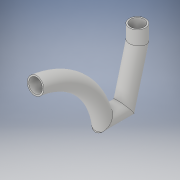
# Autodesk Inventor part: test_01
Saved by Autodesk Inventor 2019 (Build 230136000, 136)
## iProperties
Created: 2020-10-27
Part Number: test_01
Material: Genérico
Document SubType Name: Modeling
Designer: Juan M. Casillas
Density: 1 g/cm^3
Appearance: Valor por defecto
Author: Juan M. Casillas
## iProperties of the stored document test_01_3DPrint.ipt
Created: 2020-10-27
Part Number: test_01_3DPrint
Material: Genérico
Document SubType Name: Modeling
Designer: Juan M. Casillas
Density: 1 g/cm^3
Appearance: Valor por defecto
Author: Juan M. Casillas
Autodesk Inventor part; units mm, degrees
ref_plane "YZ Plane" through (0, 0, 0) normal (1, 0, 0) x (0, 1, 0)
ref_plane "XZ Plane" through (0, 0, 0) normal (0, 1, 0) x (-1, 0, 0)
ref_plane "XY Plane" through (0, 0, 0) normal (0, 0, 1) x (1, 0, 0)
sketch "Sketch7" plane through (0, 0, 0) normal (1, 0, 0) x (0, 1, 0)
  line L0 (0, 0) -> (0, 44) construction
  line L1 (0, 0) -> (44, 0) construction
  line L2 (44, 0) -> (44, 44) construction
  line L3 (44, 44) -> (0, 44) construction
  arc A0 (0, 0) -> (44, 44) centre (-6.9929, 50.9929) ccw
  line L4 (0, 0) -> (0, -22.5)
  line L5 (0, -22.5) -> (39.6996, -33.1375)
  line L6 (0, -22.5) -> (41.1, -22.5) construction
  line L7 (39.6996, -33.1375) -> (50.6736, -33.1375)
  dimension "d15" = 44
  dimension "d16" = 44
  dimension "d17" = 22.5
  dimension "d19" = 41.1
  dimension "d20" = 15
  dimension "d21" = 10.974
  constraints: 16 end point, 3 horizontal, 2 perpendicular, 2 point on circle, 2 vertical, 1 centre point, 1 equal length
  measures "d15" distance of L0.start L0.end
  measures "d16" distance of L0.start L1.end
  measures "d17" distance of L0.start L4.end
  measures "d19" distance of L4.end L5.end
  measures "d20" angle of L5 L6
  measures "d21" distance of L5.end L7.end
sketch "Sketch8" plane through (0, 0, 0) normal (0, 0, 1) x (1, 0, 0)
  line L0 (-43.2276, 7.3965) -> (-33.2276, 7.3952)
  line L1 (-33.2276, 7.3952) -> (-38.2287, -1.2644)
  line L2 (-38.2287, -1.2644) -> (-43.2276, 7.3965)
  circle A0 centre (-38.2279, 4.5091) radius 5.7817
  point P0 (0, 0)
  dimension "d18" = 10
  constraints: 6 end point, 1 centre point, 1 coincident, 7 other
  measures "d18" distance of L0.start L0.end
sweep "Sweep2" add profiles "Sketch8" path "Sketch7" path curves L7 L5 L4 A0 contours L0 L1 L2 | A0
sketch "Sketch9" plane through (-33.2276, 7.3952, -6.087) normal (0.0001268, 1, 0) x (1, -0.0001268, 0)
  line L0 (-10, 0.001) -> (0, 0) projected
  line L1 (0, 10.7385) -> (0, 0) projected
  line L2 (-10, 10.7375) -> (0, 10.7385) projected
  line L3 (-10, 10.7375) -> (-10, 0.001) projected
  point P0 (33.2285, -6.087)
extrude "Extrusion5" [suppressed]
sketch "Sketch10" plane through (-33.2276, 7.3952, -6.087) normal (0.0001268, 1, 0) x (1, -0.0001268, 0)
  line L0 (-10, 0.001) -> (0, 0) projected
  line L1 (0, 10.7385) -> (0, 0) projected
  line L2 (-10, 10.7375) -> (0, 10.7385) projected
  line L3 (-10, 10.7375) -> (-10, 0.001) projected
  point P0 (33.2285, -6.087)
extrude "Extrusion6" [suppressed]
shell "Shell4" thickness 1 removed faces 2 at (-37.9732, 50.6736, -28.5656) at (-36.8586, 49.7122, 43.2167)
chamfer "Chamfer1" [suppressed]
sketch "Sketch12" plane through (-38.2288, -1.2642, -6.0875) normal (-0.0000988, 0, 1) x (0.8660888, 0.4998902, 0.0000856)
  line L0 (0, 9.9997) -> (0, 0) projected
  line L1 (0, 9.9997) -> (-4.33, 2.4999) projected
  line L2 (0, 0) -> (-4.33, 2.4999) projected
  line L3 (0.0003, -0.0001) -> (8.6603, 4.9997) projected
  line L4 (4.3303, -2.5001) -> (0.0003, -0.0001) projected
  line L5 (8.6603, 4.9997) -> (4.3303, -2.5001) projected
  point P0 (33.742, -18.0156)
sketch "Sketch13" plane through (-38.1924, -1.2002, 1.1814) normal (-0.865962, 0.5001098, -0.0000953) x (-0.0001101, 0, 1)
  line L0 (0, 0) -> (-1.1801, 1.386) projected
  line L1 (0, 9.9258) -> (0, 0) projected
  line L2 (-8, 9.9258) -> (0, 9.9258) projected
  point P0 (-1.1856, 20.1397)
  constraints: 1 other
sketch "Sketch14" plane through (-38.2288, -1.2642, -6.8186) normal (-0.0001101, 0, 1) x (0.8660888, 0.4998902, 0.0000953)
  line L0 (0, 9.9997) -> (0, 0) projected
  line L1 (0, 9.9997) -> (-4.33, 2.4999) projected
  line L2 (0, 0) -> (-4.33, 2.4999) projected
  point P0 (33.7421, -18.0157)
sketch "Sketch16" plane through (-38.2288, -1.2642, -6.8186) normal (0.8660888, 0.4998902, 0.0000953) x (0.0001101, 0, -1)
  line L0 (-8.0829, 1.0756) -> (-6.8187, 1.4592) projected
  ellipse E0 centre (-58.2812, 0.3289) end of major axis (-8.0755, 0.3399) minor radius 43.4826 (-8.0829, 1.0756) -> (-47.1002, 42.7201) ccw projected
  line L1 (-45.172, 52.5318) -> (-47.1002, 42.7201) projected
  ellipse E1 centre (-58.2818, 2.8278) end of major axis (0.5848, 2.8408) minor radius 50.9837 (0, 9.9997) -> (-45.172, 52.5318) ccw projected
  line L2 (-8.0616, -0.0007) -> (-6.8187, 1.4592) projected
  line L3 (-8.0829, 1.0756) -> (-8.0616, -0.0007) projected
  point P0 (-6.8144, -18.0157)
  constraints: 3 other
sketch "Sketch17" plane through (-38.2288, -1.2642, -16.825) normal (-0.0000973, 0, -1) x (-0.8660888, -0.4998902, 0.0000843)
  line L0 (-8.6603, 4.9997) -> (-0.0003, -0.0001) projected
  line L1 (-8.6603, 4.9997) -> (-4.3303, -2.5001) projected
  line L2 (-0.0003, -0.0001) -> (-4.3303, -2.5001) projected
  line L3 (0, 0) -> (0, 9.9997) projected
  line L4 (4.33, 2.4999) -> (0, 0) projected
  line L5 (0, 9.9997) -> (4.33, 2.4999) projected
  point P0 (-33.7401, -18.0145)
sketch "Sketch18" plane through (-38.2282, -1.2626, -23.47) normal (-0.865962, 0.5001098, 0.0000843) x (-0.2767455, -0.4793372, 0.8328552)
  line L0 (0, 12.0047) -> (0, 0) projected
  line L1 (0, 0) -> (0.0008, -0.0012) projected
  line L2 (0.0008, -0.0016) -> (0.0008, -0.0012) projected
  line L3 (0.0008, -0.0016) -> (-28.6595, 23.3709) projected
  line L4 (-28.6595, 23.3709) -> (-23.3778, 31.0693) projected
  line L5 (-23.3778, 31.0693) -> (0, 12.0047) projected
  point P0 (8.3624, 29.8253)
sketch "Sketch19" plane through (-38.2288, -1.2642, -16.825) normal (0.8660888, 0.4998902, -0.0000843) x (-0.0000973, 0, -1)
  line L0 (6.6455, 0.0004) -> (6.645, 0.0001) projected
  line L1 (6.645, 0.0001) -> (6.6448, 0) projected
  line L2 (0, 9.9997) -> (6.6448, 0) projected
  line L3 (8.9165, 38.82) -> (0, 9.9997) projected
  line L4 (8.9165, 38.82) -> (17.5769, 35.3331) projected
  line L5 (6.6455, 0.0004) -> (17.5769, 35.3331) projected
  point P0 (-16.8287, -18.0145)
  dimension "d0" = 10
  dimension "d1" = 10
sketch "Sketch5" plane through (0, 0, 0) normal (0, 0, 1) x (1, 0, 0)
  line L0 (-5, 0) -> (5, 0)
  arc A0 (-5, 0) -> (-10.7623, 15.183) centre (-28.7327, -0.3222) ccw
  line L1 (5, 0) -> (10.4833, 17.5328)
  line L2 (10.4833, 17.5328) -> (10.4833, 24.0308)
  point P0 (0, 0)
  point P1 (0, 0)
  dimension "d11" = 10
  constraints: 6 end point, 2 point on circle, 1 centre point, 1 coincident, 1 horizontal, 1 midpoint, 1 vertical
  measures "d11" distance of L0.start L0.end
sketch "Sketch6" plane through (0, 0, 0) normal (1, 0, 0) x (0, 1, 0)
  line L0 (-2.7113, 15.3643) -> (-2.6696, 24.6845)
  line L1 (-2.6696, 24.6845) -> (5.381, 19.9883)
  line L2 (5.381, 19.9883) -> (-2.7113, 15.3643)
  point P0 (0, 0)
  point P1 (0, 20.0123)
  constraints: 6 end point, 7 other
sketch "Sketch1" plane through (0, 0, 0) normal (0, 1, 0) x (-1, 0, 0)
  line L0 (5, 5) -> (-5, 5)
  line L1 (-5, 5) -> (-5, -5)
  line L2 (-5, -5) -> (5, -5)
  line L3 (5, -5) -> (5, 5)
  line L4 (5, 5) -> (-5, -5) construction
  line L5 (-5, 5) -> (5, -5) construction
  point P0 (0, 0)
  dimension "d0" = 10
  dimension "d1" = 10
  constraints: 26 end point, 7 equal length, 4 point on line, 3 horizontal, 3 perpendicular
  measures "d0" distance of L2.end L1.end
  measures "d1" distance of L1.end L0.end
sketch "Sketch4" plane through (5, 0, 5) normal (1, 0, 0) x (0, 0, -1)
  line L0 (1, 1) -> (1, 5) projected
  line L1 (0, 5) -> (1, 5) projected
  line L2 (0, 0) -> (0, 5) projected
  line L3 (0, 0) -> (10, 0) projected
  line L4 (10, 0) -> (10, 5) projected
  line L5 (9, 5) -> (10, 5) projected
  line L6 (9, 5) -> (9, 1) projected
  line L7 (9, 1) -> (1, 1) projected
  line L8 (10, 0) -> (0, 0) projected
  line L9 (0, 1) -> (10, 1)
  line L10 (10, 1) -> (10, 0)
  line L11 (10, 0) -> (0, 0)
  line L12 (0, 0) -> (0, 1)
  point P0 (5, 0)
  constraints: 8 end point, 2 parallel, 1 horizontal, 1 perpendicular, 1 point on line
body "Solid1"
body "Solid2"
body "Solid3"
